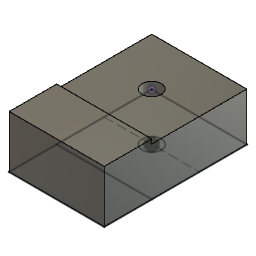
Base Plate Jig v1 (Autodesk Fusion 360 design; units mm, degrees)
Autodesk Fusion 360 part; units mm, degrees
sketch "Sketch1" plane through (0, 0, 0) normal (0, 1, 0) x (1, 0, 0)
  line L0 (0, 0) -> (20, 0)
  line L1 (20, 0) -> (20, -30)
  line L2 (20, -30) -> (0, -30)
  line L3 (0, -30) -> (0, 0)
  line L4 (0, -20) -> (20, -20)
  line L5 (0, -10) -> (20, -10) construction
  circle A0 centre (10, -10) radius 2
  dimension "d1" = 20
  dimension "d2" = 30
  dimension "d3" = 10
  dimension "d4" = 10
  dimension "d5" = 4
  constraint horizontal L0
  constraint vertical L1
  constraint horizontal L2
  constraint vertical L3
  constraint coincident L0.start L3.end
  constraint coincident L3 L4.start
  constraint coincident L1 L4.end
  constraint perpendicular L1 L4
  constraint coincident L3 L5.start
  constraint coincident L1 L5.end
  constraint perpendicular L1 L5
  constraint midpoint L5 A0.centre
  measures "d1" distance of L0.start L0.end
  measures "d2" distance of L0.start L2.end
  measures "d3" distance of L2 L4
  measures "d4" distance of L0 L5
  measures "d5" diameter of A0
extrude "Extrude1" add sketch "Sketch1" along normal blind 11 contours L1 L2 L3 L4
extrude "Extrude2" add sketch "Sketch1" along normal blind 10.0856 contours L0 L1 L3 L4
equation "d8 = 11 mm - 0.036 in"
named bodies: "Base Plate Jig"
